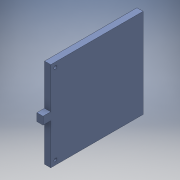
# Autodesk Inventor part: extremite_pince
Saved by Autodesk Inventor 2017 SP1 (Build 210196100, 196)
## iProperties
Created: 2017-11-21
Part Number: extremite_pince
Material: PC/ABS Plastic
Document SubType Name: Modeling
Designer: Biscuit
Density: 0.357273 g/cm^3
Appearance: Rubber - Blue
Author: Biscuit
Autodesk Inventor part; units mm, degrees
ref_plane "YZ Plane" through (0, 0, 0) normal (1, 0, 0) x (0, 1, 0)
ref_plane "XZ Plane" through (0, 0, 0) normal (0, 1, 0) x (-1, 0, 0)
ref_plane "XY Plane" through (0, 0, 0) normal (0, 0, 1) x (1, 0, 0)
sketch "Sketch1" plane through (0, 0, 0) normal (0, 1, 0) x (-1, 0, 0)
  line L0 (0, 0) -> (4, 0)
  line L1 (4, 0) -> (4, -58)
  line L2 (4, -58) -> (0, -58)
  line L3 (0, -58) -> (0, 0)
  dimension "d0" = 58
  dimension "d1" = 4
  constraints: 8 end point, 2 parallel, 1 horizontal, 1 perpendicular
  measures "d0" distance of L0.end L1.end
  measures "d1" distance of L1.end L2.end
extrude "Extrusion1" add sketch "Sketch1" along normal blind 60
sketch "Sketch2" plane through (-4, 0, 0) normal (0, 0, 1) x (1, 0, 0)
  circle A0 centre (2, 2) radius 1
  line L0 (4, 0) -> (0, 0) projected
  line L1 (4, 0) -> (4, 60) projected
  dimension "d4" = 2
  dimension "d5" = 2
  dimension "d6" = 2
  constraints: 1 centre point
  measures "d4" diameter of A0
  measures "d5" distance from line of L0 A0.centre
  measures "d6" distance from line of L1 A0.centre
extrude "Extrusion2" [suppressed]
fillet "Fillet1" [suppressed]
sketch "Sketch3" plane through (0, 2, 0) normal (1, 0, 0) x (0, 0, -1)
  line L0 (19, 20.5) -> (24, 20.5)
  line L1 (24, 20.5) -> (24, 35.5)
  line L2 (24, 35.5) -> (19, 35.5)
  line L3 (19, 35.5) -> (19, 20.5)
  line L4 (34, 20.5) -> (39, 20.5)
  line L5 (39, 20.5) -> (39, 35.5)
  line L6 (39, 35.5) -> (34, 35.5)
  line L7 (34, 35.5) -> (34, 20.5)
  line L8 (0, -2) -> (0, 58) projected
  line L9 (58, -2) -> (58, 58) projected
  line L10 (0, -2) -> (58, -2) projected
  line L11 (0, 58) -> (58, 58) projected
  point P0 (0, 0)
  point P1 (0, 56)
  point P2 (58, 0)
  point P3 (58, 56)
  dimension "d10" = 15
  dimension "d11" = 15
  dimension "d12" = 5
  dimension "d13" = 5
  dimension "d14" = 10
  dimension "d15" = 19
  dimension "d16" = 58
  dimension "d17" = 60
  dimension "d18" = 22.5
  constraints: 16 end point, 4 parallel, 2 horizontal, 2 perpendicular, 1 point on line
  measures "d10" distance of L2.end L0.start
  measures "d11" distance of L6.end L4.start
  measures "d12" distance of L0.start L0.end
  measures "d13" distance of L4.start L4.end
  measures "d14" distance between parallel lines of L7 L1
  measures "d15" distance between parallel lines of L8 L3
  measures "d16" distance between parallel lines of L9 L8
  measures "d17" distance between parallel lines of L11 L10
  measures "d18" distance between parallel lines of L10 L0
extrude "Extrusion3" [suppressed]
sketch "Sketch4" plane through (0, 22.5, -19) normal (0, 0, 1) x (1, 0, 0)
  circle A0 centre (5, 7.5) radius 1.5
  line L0 (0, 0) -> (10, 0) projected
  line L1 (10, 0) -> (10, 15) projected
  point P0 (0, -22.5)
  dimension "d21" = 3
  dimension "d22" = 7.5
  dimension "d23" = 5
  dimension "d24" = 15
  dimension "d25" = 10
  constraints: 1 centre point
  measures "d21" diameter of A0
  measures "d22" distance from line of L0 A0.centre
  measures "d23" distance from line of L1 A0.centre
  measures "d24" distance of L0.end L1.end
  measures "d25" distance of L0.start L0.end
extrude "Extrusion4" [suppressed]
fillet "Fillet2" [suppressed]
sketch "Esquisse5" plane through (0, 0, 0) normal (1, 0, 0) x (0, 0, -1)
  circle A0 centre (55, 3) radius 1
  circle A1 centre (3, 3) radius 1
  line L0 (0, 0) -> (0, 60) projected
  line L1 (58, 0) -> (0, 0) projected
  line L2 (58, 0) -> (58, 60) projected
  dimension "d29" = 2
  dimension "d30" = 2
  dimension "d31" = 3
  dimension "d32" = 3
  dimension "d33" = 3
  dimension "d34" = 3
  constraints: 2 centre point
  measures "d29" diameter of A0
  measures "d30" diameter of A1
  measures "d31" distance from line of L0 A1.centre
  measures "d32" distance from line of L1 A1.centre
  measures "d33" distance from line of L2 A0.centre
  measures "d34" distance from line of L1 A0.centre
extrude "Extrusion5" cut sketch "Esquisse5" against normal blind 10
sketch "Esquisse6" plane through (0, 0, 0) normal (0, -1, 0) x (1, 0, 0)
  line L0 (-4, -58) -> (-4, 0) projected
  line L1 (0, 0) -> (0, -58) projected
  line L2 (-4, -26.5) -> (0, -26.5)
  line L3 (0, -26.5) -> (0, -31.5)
  line L4 (0, -31.5) -> (-4, -31.5)
  line L5 (-4, -31.5) -> (-4, -26.5)
  line L6 (0, 0) -> (-4, 0) projected
  dimension "d37" = 5
  dimension "d38" = 26.5
  dimension "d39" = 58
  constraints: 8 end point, 2 parallel, 2 point on line, 1 horizontal, 1 perpendicular
  measures "d37" distance between parallel lines of L2 L4
  measures "d38" distance between parallel lines of L6 L2
  measures "d39" distance of L0.start L0.end
extrude "Extrusion6" add sketch "Esquisse6" along normal blind 5 contours L0 L2 L1 L4
equation "\"d6\" = d5"
equation "\"d11\" = d10"
equation "\"d13\" = d12"
equation "\"d15\" = 0.5 * d16 - 0.5 * d14 - 0.5 * d12 - 0.5 * d13"
equation "\"d18\" = 0.5 * d17 - 0.5 * d10"
equation "\"d22\" = 0.5 * d24"
equation "\"d23\" = 0.5 * d25"
equation "\"d32\" = d31"
equation "\"d33\" = d32"
equation "\"d34\" = d33"
equation "\"d38\" = 0.5 * d39 - 0.5 * d37"
body "Solid1"
